Untitled (Autodesk Fusion 360 design; units mm, degrees)
Autodesk Fusion 360 part; units mm, degrees
sketch "Sketch1" plane through (0, 0, 0) normal (0, 1, 0) x (1, 0, 0)
  line L0 (0, 64.0421) -> (0, -79.964)
  line L1 (-3.05, -8) -> (-3.05, 0)
  line L2 (-6.25, 0) -> (-6.25, 12)
  line L3 (-6.25, 0) -> (-3.05, 0)
  line L4 (-8.05, -8) -> (-8.05, -5)
  line L5 (-11.25, -5) -> (-8.05, -5)
  line L6 (-11.25, -5) -> (-11.25, 12)
  line L7 (-8.05, -8) -> (-3.05, -8)
  line L8 (-11.25, 12) -> (-6.25, 12)
  line L9 (-3.05, -8) -> (0, -7.961)
  line L10 (-6.25, 12) -> (0, 12)
  dimension "d1" = 12.5
  dimension "d2" = 6.1
  dimension "d3" = 8
  dimension "d7" = 12
  dimension "d8" = -5
  constraint vertical L0
  constraint parallel L0 L1
  constraint coincident origin L0
  constraint collinear origin L1.end L2.start
  constraint horizontal L3
  constraint perpendicular L2 L8
  constraint midpoint L0 L9.end
  constraint coincident L0 L10.end
  constraint perpendicular L0 L10
  measures "d3" distance of L1.start L1.end
  measures "d7" distance of L2.start L2.end
revolve "Revolve1" add sketch "Sketch1" angle 360 about axis through (0, 0, -64.0421) along (0, 0, 1)
sketch "Sketch2" plane through (0, 0, 8) normal (0, 0, 1) x (-1, 0, 0)
  circle A0 centre (0, 0) radius 3.05 construction
  circle A1 centre (0, 0) radius 8.05
  line L0 (-3.05, 3.05) -> (3.05, 3.05)
  line L1 (3.05, 3.05) -> (3.05, -3.05)
  line L2 (3.05, -3.05) -> (-3.05, -3.05)
  line L3 (-3.05, -3.05) -> (-3.05, 3.05)
  line L4 (-3.05, 3.05) -> (3.05, -3.05) construction
  line L5 (3.05, 3.05) -> (-3.05, -3.05) construction
  point P0 (3.05, 0)
  constraint horizontal L0
  constraint perpendicular L0 L1
  constraint parallel L0 L2
  constraint parallel L1 L3
  constraint coincident L4 A0.centre
  constraint coincident L5 A0.centre
  constraint coincident A0.centre A1.centre
  constraint tangent A0 L0
  constraint tangent A0 L3
extrude "Extrude1" cut sketch "Sketch2" against normal through all contours L0 L1 L2 L3
sketch "Sketch3" plane through (0, 0, -12) normal (0, 0, -1) x (1, 0, 0)
  line L0 (3.05, 3.05) -> (3.05, -3.05)
  line L1 (3.05, -3.05) -> (-3.05, -3.05)
  line L2 (-3.05, -3.05) -> (-3.05, 3.05)
  line L3 (-3.05, 3.05) -> (3.05, 3.05)
  circle A0 centre (0, 0) radius 11.25
  line L4 (-6, 6) -> (6, 6)
  line L5 (6, 6) -> (6, -6)
  line L6 (6, -6) -> (-6, -6)
  line L7 (-6, -6) -> (-6, 6)
  line L8 (-6, 6) -> (6, -6) construction
  line L9 (6, 6) -> (-6, -6) construction
  dimension "d11" = 12
  dimension "d12" = 12
  constraint horizontal L4
  constraint perpendicular L4 L5
  constraint parallel L4 L6
  constraint parallel L5 L7
  constraint coincident L8 A0.centre
  constraint coincident L9 A0.centre
  constraint coincident A0.centre origin
  measures "d11" distance of L5.end L6.end
  measures "d12" distance of L4.end L5.end
extrude "Extrude2" cut sketch "Sketch3" against normal blind 12 contours L4 L5 L6 L7
chamfer "Chamfer1" distance 1.9 angle 45 1 edges at (-7.5052, 2.911, 5)
